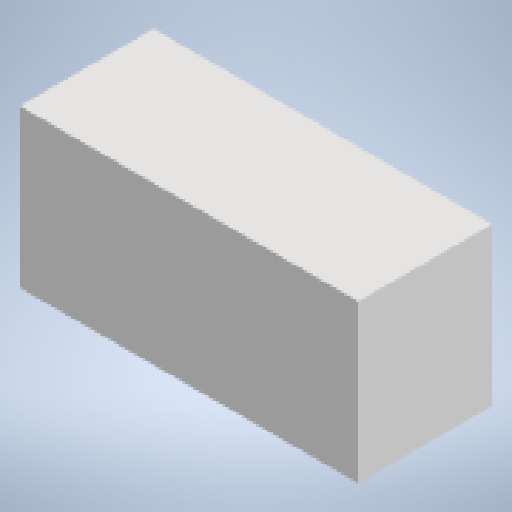
# Autodesk Inventor part: WPC_Asztal_200x100
Saved by Autodesk Inventor 2025.2 (Build 292293000, 293)
## iProperties
Created: 2025-03-10
Part Number: WPC_Asztal_200x100
Material: Generic
Document SubType Name: Modeling
Designer: MB
Density: 1 g/cm^3
Appearance: Default
Author: MB
Autodesk Inventor part; units mm, degrees
ref_plane "YZ Plane" through (0, 0, 0) normal (1, 0, 0) x (0, 1, 0)
ref_plane "XZ Plane" through (0, 0, 0) normal (0, 1, 0) x (-1, 0, 0)
ref_plane "XY Plane" through (0, 0, 0) normal (0, 0, 1) x (1, 0, 0)
sketch "Sketch1" plane through (0, 0, 0) normal (0, 0, 1) x (1, 0, 0)
  line L0 (0, 0) -> (2000, 0)
  line L1 (2000, 0) -> (2000, 1000)
  line L2 (2000, 1000) -> (0, 1000)
  line L3 (0, 1000) -> (0, 0)
  dimension "d0" = 2000
  dimension "d1" = 1000
  constraints: 8 end point, 2 parallel, 1 horizontal, 1 perpendicular
  measures "d0" distance of L2.end L1.end
  measures "d1" distance of L1.end L0.end
extrude "Extrusion1" add sketch "Sketch1" along normal blind 850
sketch "Sketch3" plane through (0, 0, 850) normal (0, 0, 1) x (1, 0, 0)
  line L0 (2000, 0) -> (2000, 1000) construction
  line L1 (2000, 1000) -> (0, 1000) construction
  line L2 (0, 1000) -> (0, 0) construction
  line L3 (0, 0) -> (2000, 0) construction
  line L4 (500, 1000) -> (500, 0)
  line L5 (0, 0) -> (2000, 0) construction
  line L6 (1000, 1000) -> (1000, 0)
  line L7 (1500, 1000) -> (1500, 0)
  line L8 (0, 1000) -> (2000, 1000)
  line L9 (2000, 1000) -> (2000, 0)
  line L10 (0, 0) -> (2000, 0)
  line L11 (0, 1000) -> (0, 0)
  dimension "d5" = 500
  dimension "d8" = 500
  constraints: 14 end point, 4 collinear, 2 point on line, 1 horizontal, 1 perpendicular, 6 other
  measures "d5" distance between parallel lines of L2 L4
  measures "d8" distance of L4.start L6.start
body "Solid1"
